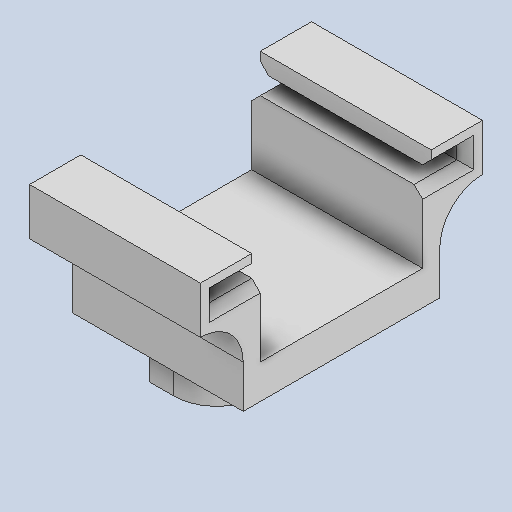
# Autodesk Inventor part: Drziak_3
Saved by Autodesk Inventor 2025 (Build 290162000, 162)
## iProperties
Created: 2025-06-09
Part Number: Drziak_3
Material: Generic
Document SubType Name: Modeling
Designer: Pravoslav
Density: 1 g/cm^3
Appearance: Default
Author: Pravoslav
Autodesk Inventor part; units mm, degrees
ref_plane "YZ Plane" through (0, 0, 0) normal (1, 0, 0) x (0, 1, 0)
ref_plane "XZ Plane" through (0, 0, 0) normal (0, 1, 0) x (-1, 0, 0)
ref_plane "XY Plane" through (0, 0, 0) normal (0, 0, 1) x (1, 0, 0)
sketch "Sketch1" plane through (0, 0, 0) normal (1, 0, 0) x (0, 1, 0)
  line L0 (0, 9.5) -> (0, -9.5)
  line L1 (0, -9.5) -> (8, -9.5)
  line L2 (0, 9.5) -> (8, 9.5)
  line L3 (8, 9.5) -> (8, 14.5)
  line L4 (8, 14.5) -> (9.5, 14.5)
  line L5 (9.5, 14.5) -> (9.5, 10.5)
  line L6 (9.5, 10.5) -> (11.5, 10.5)
  line L7 (11.5, 10.5) -> (11.5, 16.5)
  line L8 (11.5, 16.5) -> (6, 16.5)
  line L9 (6, 16.5) -> (6, 11.5)
  line L10 (6, 11.5) -> (-3, 11.5)
  line L11 (-3, 11.5) -> (-4, 11.5)
  line L12 (-4, 11.5) -> (-4, 1)
  line L13 (0, 0) -> (3.5, 0)
  line L14 (0, -9.5) -> (8, -9.5)
  line L15 (8, -9.5) -> (8, -14.5)
  line L16 (8, -14.5) -> (9.5, -14.5)
  line L17 (9.5, -14.5) -> (9.5, -10.5)
  line L18 (11.5, -10.5) -> (11.5, -16.5)
  line L19 (11.5, -16.5) -> (6, -16.5)
  line L20 (6, -16.5) -> (6, -11.5)
  line L21 (6, -11.5) -> (-3, -11.5)
  line L22 (-3, -11.5) -> (-4, -11.5)
  line L23 (-4, -11.5) -> (-4, 1)
  line L24 (11.5, -10.5) -> (9.5, -10.5)
  point P0 (8.75, -16.5)
  point P1 (8.75, -14.5)
  dimension "d0" = 19
  dimension "d1" = 0
  dimension "d2" = 8
  dimension "d3" = 8
  dimension "d4" = 5
  dimension "d5" = 1.5
  dimension "d6" = 2
  dimension "d7" = 6
  dimension "d8" = 5.5
  dimension "d9" = 5
  dimension "d10" = 1
  dimension "d13" = 2
  dimension "d14" = 4
  constraints: 50 end point, 9 symmetric about line, 8 perpendicular, 4 horizontal, 3 midpoint, 2 point on line, 2 vertical
  measures "d0" distance of L0.start L0.end
  measures "d1" distance of point (0, 0) L13.start
  measures "d2" distance of L0.end L1.end
  measures "d3" distance of L0.start L2.end
  measures "d4" distance of L2.end L3.end
  measures "d5" distance of L3.end L4.end
  measures "d6" distance of L5.end L6.end
  measures "d7" distance of L6.end L7.end
  measures "d8" distance of L7.end L8.end
  measures "d9" distance of L8.end L9.end
  measures "d10" distance of L10.end L11.end
  measures "d13" distance of point (8.75, -16.5) point (8.75, -14.5)
  measures "d14" distance between parallel lines of L23 L0
extrude "Extrusion1" add sketch "Sketch1" along normal blind 20
fillet "Fillet1" radius 5 2 edges at (10, 6, -11.5) (10, 6, 11.5)
chamfer "Chamfer1" distance 1 angle 45 12 edges at (20, 8, -12) (20, 8.75, -14.5) (20, 9.5, -12.5) (20, 8, 12) (20, 8.75, 14.5) (20, 9.5, 12.5) (0, 8, -12) (0, 8.75, -14.5) (0, 9.5, -12.5) (0, 8, 12) (0, 8.75, 14.5) (0, 9.5, 12.5)
sketch "Sketch3" plane through (0, -4, -11.5) normal (0, -1, 0) x (1, 0, 0)
  line L0 (6, 15.5002) -> (13.9, 15.5002)
  line L1 (13.9, 15.5002) -> (13.9, 7.6002)
  line L2 (13.9, 7.6002) -> (6, 7.6002)
  line L3 (6, 7.6002) -> (6, 15.5002)
  line L4 (0, 23) -> (0, 0) projected
  line L5 (0, 23) -> (20, 23) projected
  point P0 (0, 11.5)
  point P1 (10, 23)
  point P2 (9.95, 15.5002)
  dimension "d27" = 7.9
  dimension "d28" = 7.9
  dimension "d29" = 6
  dimension "d30" = 7.5
  constraints: 8 end point, 2 midpoint, 2 parallel, 1 horizontal, 1 perpendicular
  measures "d27" distance of L1.end L2.end
  measures "d28" distance of L0.end L1.end
  measures "d29" distance between parallel lines of L4 L3
  measures "d30" distance of point (10, 23) point (9.95, 15.5)
extrude "Extrusion3" add sketch "Sketch3" along normal blind 2.5
sketch "Sketch4" plane through (0, -6.5, -11.5) normal (0, -1, 0) x (1, 0, 0)
  line L0 (13.9, 3.1002) -> (6, 3.1002)
  line L1 (6, 3.1002) -> (6, 20.0002)
  line L2 (6, 20.0002) -> (13.9, 20.0002)
  line L3 (13.9, 20.0002) -> (13.9, 3.1002)
  line L4 (13.9, 3.1002) -> (6, 20.0002) construction
  line L5 (6, 3.1002) -> (13.9, 20.0002) construction
  line L6 (6, 15.5002) -> (6, 7.6002) projected
  line L7 (6, 7.6002) -> (13.9, 7.6002) projected
  point P0 (0, 11.5)
  point P1 (9.95, 11.5502)
  dimension "d33" = 7.9
  dimension "d34" = 16.9
  dimension "d35" = 0
  dimension "d36" = 4.5
  constraints: 12 end point, 2 midpoint, 2 parallel, 1 horizontal, 1 perpendicular
  measures "d33" distance of L1.end L2.end
  measures "d34" distance of L0.end L1.end
  measures "d35" distance between parallel lines of L6 L1
  measures "d36" distance between parallel lines of L7 L0
extrude "Extrusion4" add sketch "Sketch4" along normal blind 3
fillet "Fillet2" radius 5 4 edges at (6, -5.25, -3.8998) (6, -8, -8.3998) (13.9, -5.25, 4.0002) (13.9, -8, 8.5002)
sketch "Sketch2" plane through (0, 0, 9.5) normal (0, 1, 0) x (1, 0, 0)
  circle A0 centre (10, 9.5) radius 3
  line L0 (20, 19) -> (20, 0) projected
  line L1 (0, -7) -> (20, -7) projected
  point P0 (0, 9.5)
  dimension "d19" = 6
  dimension "d20" = 10
  dimension "d21" = 16.5
  constraints: 1 centre point
  measures "d19" diameter of A0
  measures "d20" distance from line of L0 A0.centre
  measures "d21" distance from line of L1 A0.centre
body "Solid1"
